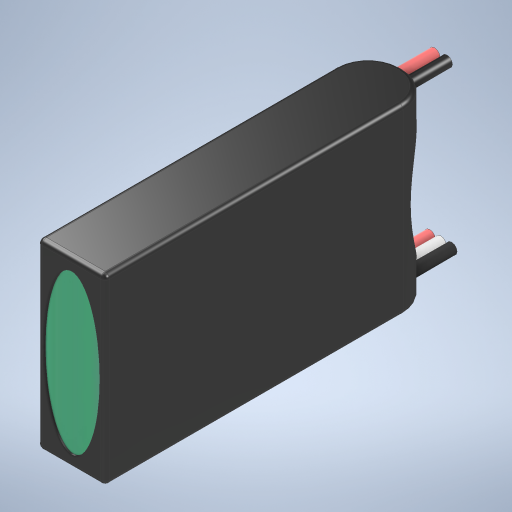
# Autodesk Inventor part: 2s Driving Battery
Saved by Autodesk Inventor 2024 (Build 280153000, 153)
## iProperties
Created: 2023-11-10
Part Number: 2s Driving Battery
Material: Generic
Document SubType Name: Modeling
Designer: 18179
Density: 1 g/cm^3
Appearance: Default
Author: 18179
Autodesk Inventor part; units mm, degrees
ref_plane "YZ Plane" through (0, 0, 0) normal (1, 0, 0) x (0, 1, 0)
ref_plane "XZ Plane" through (0, 0, 0) normal (0, 1, 0) x (-1, 0, 0)
ref_plane "XY Plane" through (0, 0, 0) normal (0, 0, 1) x (1, 0, 0)
sketch "Sketch1" plane through (0, 0, 0) normal (0, 0, 1) x (1, 0, 0)
  line L0 (0, 0) -> (11.049, 0)
  line L1 (11.049, 0) -> (11.049, 29.845)
  line L2 (11.049, 29.845) -> (0, 29.845)
  line L3 (0, 29.845) -> (0, 0)
  dimension "d0" = 11.049
  dimension "d1" = 29.845
  constraints: 8 end point, 2 parallel, 1 horizontal, 1 perpendicular
  measures "d0" distance of L2.end L1.end
  measures "d1" distance of L1.end L0.end
extrude "Extrusion1" add sketch "Sketch1" against normal blind 53.9369
fillet "Fillet1" radius 5.334 2 edges at (11.049, 14.9225, -53.9369) (0, 14.9225, -53.9369)
sketch "Sketch2" plane through (11.049, 0, 0) normal (1, 0, 0) x (0, 0, -1)
  line L0 (53.9369, 29.845) -> (53.9369, 26.67)
  line L1 (53.9369, 29.845) -> (53.9369, 0) projected
  line L2 (53.9369, 0) -> (53.9369, 3.175)
  arc A0 (53.9369, 26.67) -> (53.9369, 3.175) centre (69.6154, 14.9225) ccw
  point P0 (0, 0)
  dimension "d5" = 3.175
  dimension "d6" = 3.175
  constraints: 4 end point, 2 point on circle, 2 point on line, 1 centre point
  measures "d5" distance of L0.start L0.end
  measures "d6" distance of L1.end L2.end
extrude "Extrusion2" cut sketch "Sketch2" against normal blind 53.9369
sketch "Sketch3" plane through (0, 0, -53.9369) normal (0, 0, -1) x (-1, 0, 0)
  spline S0 degree 5 poles (-5.715, 3.175) (-6.1097, 3.175) (-6.5044, 3.2237) (-6.8883, 3.3211) (-7.253, 3.4636) (-8.0021, 3.8637) (-8.3758, 4.1396) (-8.7032, 4.4603) (-8.9888, 4.8153) (-9.6114, 5.7716) (-9.8983, 6.4056) (-10.116, 7.0698) (-10.2843, 7.7518) (-10.65, 9.6976) (-10.7645, 10.9938) (-10.8259, 12.2987) (-10.8562, 13.6081) (-10.8562, 16.3635) (-10.8199, 17.7955) (-10.7459, 19.2233) (-10.6035, 20.6422) (-10.2134, 22.3259) (-10.1252, 22.6569) (-10.0247, 22.983) (-9.9101, 23.3028) (-9.6124, 24.0099) (-9.419, 24.3934) (-9.1943, 24.7587) (-8.9346, 25.0991) (-8.4946, 25.5536) (-8.3445, 25.6923) (-8.186, 25.8226) (-8.0193, 25.9433) (-7.4721, 26.2884) (-7.0628, 26.4761) (-6.6247, 26.6053) (-6.1699, 26.67) (-5.715, 26.67) knots 0 0 0 0 0 0 0.067999 0.067999 0.067999 0.067999 0.150178 0.150178 0.150178 0.150178 0.275142 0.275142 0.275142 0.275142 0.499815 0.499815 0.499815 0.499815 0.746132 0.746132 0.746132 0.746132 0.807282 0.807282 0.807282 0.807282 0.884858 0.884858 0.884858 0.884858 0.921632 0.921632 0.921632 0.921632 1 1 1 1 1 1 projected
  line L0 (-5.334, 3.175) -> (-5.715, 3.175) projected
  spline S1 degree 5 poles (-5.334, 26.67) (-4.8791, 26.67) (-4.4243, 26.6053) (-3.9862, 26.4761) (-3.5769, 26.2884) (-3.0297, 25.9433) (-2.863, 25.8226) (-2.7045, 25.6923) (-2.5544, 25.5536) (-2.1144, 25.0991) (-1.8547, 24.7587) (-1.63, 24.3934) (-1.4366, 24.0099) (-1.1389, 23.3028) (-1.0243, 22.983) (-0.9238, 22.6569) (-0.8356, 22.3259) (-0.4455, 20.6422) (-0.3031, 19.2233) (-0.2291, 17.7955) (-0.1928, 16.3635) (-0.1928, 13.6081) (-0.2231, 12.2987) (-0.2845, 10.9938) (-0.399, 9.6976) (-0.7647, 7.7518) (-0.933, 7.0698) (-1.1507, 6.4056) (-1.4376, 5.7716) (-2.0602, 4.8153) (-2.3458, 4.4603) (-2.6732, 4.1396) (-3.0469, 3.8637) (-3.796, 3.4636) (-4.1607, 3.3211) (-4.5446, 3.2237) (-4.9393, 3.175) (-5.334, 3.175) knots 0 0 0 0 0 0 0.078368 0.078368 0.078368 0.078368 0.115142 0.115142 0.115142 0.115142 0.192718 0.192718 0.192718 0.192718 0.253868 0.253868 0.253868 0.253868 0.500185 0.500185 0.500185 0.500185 0.724858 0.724858 0.724858 0.724858 0.849822 0.849822 0.849822 0.849822 0.932001 0.932001 0.932001 0.932001 1 1 1 1 1 1 projected
  line L1 (-5.715, 26.67) -> (-5.334, 26.67) projected
  point P0 (0, 0)
  constraints: 2 vertical alignment
extrude "Extrusion3" cut sketch "Sketch3" against normal blind 5.08
fillet "Fillet2" radius 0.762 14 edges at (9.4867, 29.845, -52.3746) (5.5245, 29.845, -53.9369) (1.5623, 29.845, -52.3746) (0, 29.845, -24.3015) (11.049, 29.845, -24.3015) (5.5245, 29.845, 0) (11.049, 14.9225, 0) (0, 14.9225, 0) (5.5245, 0, 0) (9.4867, 0, -52.3746) (5.5245, 0, -53.9369) (1.5623, 0, -52.3746) (0, 0, -24.3015) (11.049, 0, -24.3015)
sketch "Sketch4" plane through (0, 0, 0) normal (0, 0, 1) x (1, 0, 0)
  line L0 (10.287, 29.083) -> (10.287, 0.762) projected
  line L1 (0.762, 29.083) -> (10.287, 29.083) projected
  line L2 (0.762, 0.762) -> (0.762, 29.083) projected
  line L3 (10.287, 0.762) -> (0.762, 0.762) projected
  ellipse E0 centre (5.6197, 14.9232) end of major axis (5.6197, 27.8786) minor radius 4.5697
  line L4 (5.6197, 14.9232) -> (5.6197, 1.9678)
  point P0 (0, 0)
  constraints: 2 end point, 2 vertical, 1 vertical alignment, 2 other
extrude "Extrusion4" cut sketch "Sketch4" against normal blind 0.254 contours E0
sketch "Sketch5" plane through (0, 0, -53.9369) normal (0, 0, -1) x (-1, 0, 0)
  line L0 (-5.715, 26.67) -> (-5.334, 26.67) projected
  line L1 (-5.5245, 26.67) -> (-5.5245, 27.8765)
  line L2 (-5.5245, 27.8765) -> (-4.5085, 27.8765)
  line L3 (-5.5245, 27.8765) -> (-6.5405, 27.8765)
  circle A0 centre (-6.5405, 27.8765) radius 0.889
  circle A1 centre (-4.5085, 27.8765) radius 0.889
  line L4 (-5.334, 3.175) -> (-5.715, 3.175) projected
  line L5 (-5.5245, 3.175) -> (-5.5245, 1.8135)
  circle A2 centre (-5.5245, 1.8135) radius 0.889
  line L6 (-5.5245, 1.8135) -> (-3.7465, 1.8135)
  line L7 (-3.7465, 1.8135) -> (-7.3025, 1.8135)
  circle A3 centre (-7.3025, 1.8135) radius 0.889
  circle A4 centre (-3.7465, 1.8135) radius 0.889
  point P0 (0, 0)
  point P1 (-6.4135, 1.8135)
  point P2 (-4.6355, 1.8135)
  dimension "d14" = 1.016
  dimension "d15" = 1.778
  dimension "d16" = 1.778
  dimension "d17" = 1.016
  dimension "d18" = 1.778
  dimension "d19" = 1.778
  dimension "d20" = 3.556
  constraints: 12 end point, 5 centre point, 5 coincident, 2 midpoint, 2 point on line, 2 vertical, 1 horizontal, 1 perpendicular
  measures "d14" distance of L1.end L3.end
  measures "d15" diameter of A0
  measures "d16" diameter of A1
  measures "d17" distance of L1.end L2.end
  measures "d18" diameter of A2
  measures "d19" distance of L6.start L6.end
  measures "d20" distance of L6.end L7.end
extrude "Extrusion5" add sketch "Sketch5" along normal blind 6.35 and the other way blind 2.54
sketch "Sketch6" plane through (0, 0.762, -0.762) normal (-1, 0, 0) x (0, 0, 1)
  line L0 (-48.0478, 25.9916) -> (-1.0689, 25.9916) construction
  line L1 (-1.0689, 25.9916) -> (-1.0689, 2.2942) construction
  line L2 (-1.0689, 2.2942) -> (-48.0478, 2.2942) construction
  line L3 (-48.0478, 2.2942) -> (-48.0478, 25.9916) construction
  point P0 (0.762, -0.762)
  constraints: 2 other
decal "Decal1"
body "Solid1"
